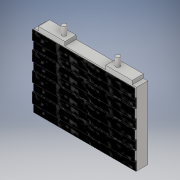
# Autodesk Inventor part: Cell
Saved by Autodesk Inventor 2017 (Build 210142000, 142)
## iProperties
Created: 2021-02-12
Part Number: Cell
Material: Generic
Document SubType Name: Modeling
Designer: Win240
Density: 1 g/cm^3
Appearance: Default
Author: Win240
Autodesk Inventor part; units mm, degrees
ref_plane "YZ Plane" through (0, 0, 0) normal (1, 0, 0) x (0, 1, 0)
ref_plane "XZ Plane" through (0, 0, 0) normal (0, 1, 0) x (-1, 0, 0)
ref_plane "XY Plane" through (0, 0, 0) normal (0, 0, 1) x (1, 0, 0)
sketch "Sketch1" plane through (0, 0, 0) normal (0, 0, 1) x (1, 0, 0)
  line L0 (-60.325, -42.8625) -> (60.325, -42.8625)
  line L1 (60.325, -42.8625) -> (60.325, 42.8625)
  line L2 (60.325, 42.8625) -> (-60.325, 42.8625)
  line L3 (-60.325, 42.8625) -> (-60.325, -42.8625)
  line L4 (-60.325, -42.8625) -> (60.325, 42.8625) construction
  line L5 (60.325, -42.8625) -> (-60.325, 42.8625) construction
  line L6 (-55.245, 42.8625) -> (-55.245, 47.3075)
  line L7 (-55.245, 47.3075) -> (-24.13, 47.3075)
  line L8 (-24.13, 47.3075) -> (-24.13, 42.8625)
  line L9 (24.13, 42.8625) -> (24.13, 47.3075)
  line L10 (24.13, 47.3075) -> (55.245, 47.3075)
  line L11 (55.245, 47.3075) -> (55.245, 42.8625)
  point P0 (0, 0)
  dimension "d0" = 120.65
  dimension "d1" = 85.725
  dimension "d2" = 4.445
  dimension "d3" = 5.08
  dimension "d4" = 5.08
  dimension "d5" = 31.115
  constraints: 24 end point, 4 point on line, 4 vertical, 2 collinear, 2 horizontal, 2 midpoint, 2 parallel, 1 perpendicular
  measures "d0" distance of L1.end L2.end
  measures "d1" distance of L2.end L0.start
  measures "d2" distance between parallel lines of L7 L2
  measures "d3" distance between parallel lines of L6 L3
  measures "d4" distance between parallel lines of L1 L11
  measures "d5" distance of L9.end L10.end
extrude "Extrusion1" add sketch "Sketch1" along normal blind 13.335
ref_plane "Work Plane1" through (-60.325, 57.1375, 0) normal (0, -1, 0) x (1, 0, 0)
sketch "Sketch2" plane through (-55.245, 47.3075, 0) normal (0, 1, 0) x (1, 0, 0)
  line L0 (31.115, 0) -> (31.115, -13.335) construction
  line L1 (79.375, 0) -> (79.375, -13.335) construction
  line L2 (31.115, -6.6675) -> (23.495, -6.6675) construction
  line L3 (79.375, -6.6675) -> (86.995, -6.6675) construction
  circle A0 centre (23.495, -6.6675) radius 2.5
  circle A1 centre (86.995, -6.6675) radius 2.5
  point P0 (55.245, 0)
  dimension "d8" = 63.5
  dimension "d9" = 5
  constraints: 4 end point, 2 centre point, 2 coincident, 2 horizontal, 2 midpoint, 1 collinear, 1 equal radius
  measures "d8" distance of L3.end L2.end
  measures "d9" diameter of A1
extrude "Extrusion2" add sketch "Sketch2" along normal up to surface (9.83 mm away)
sketch "Sketch3" plane through (60.325, -42.8625, 0) normal (1, 0, 0) x (0, 0, -1)
  line L0 (0, 0) -> (-13.335, 0) construction
  line L1 (-13.335, 0) -> (-13.335, 10.7156)
  line L2 (-13.335, 10.7156) -> (-14.985, 10.7156)
  line L3 (-14.985, 10.7156) -> (-14.985, 21.4313)
  line L4 (-14.985, 21.4313) -> (-13.335, 21.4313)
  line L5 (-13.335, 21.4313) -> (-13.335, 32.1469)
  line L6 (-13.335, 32.1469) -> (-14.985, 32.1469)
  line L7 (-14.985, 32.1469) -> (-14.985, 42.8625)
  line L8 (-14.985, 42.8625) -> (-13.335, 42.8625)
  line L9 (-13.335, 42.8625) -> (-13.335, 53.5781)
  line L10 (-13.335, 53.5781) -> (-14.985, 53.5781)
  line L11 (-14.985, 53.5781) -> (-14.985, 64.2938)
  line L12 (-14.985, 64.2938) -> (-13.335, 64.2938)
  line L13 (-13.335, 64.2938) -> (-13.335, 75.0094)
  line L14 (-13.335, 75.0094) -> (-14.985, 75.0094)
  line L15 (-14.985, 75.0094) -> (-14.985, 85.725)
  line L16 (-15.585, 85.725) -> (-15.585, 74.4094)
  line L17 (-15.585, 74.4094) -> (-13.935, 74.4094)
  line L18 (-13.935, 74.4094) -> (-13.935, 64.8938)
  line L19 (-13.935, 64.8938) -> (-15.585, 64.8938)
  line L20 (-15.585, 64.8938) -> (-15.585, 52.9781)
  line L21 (-15.585, 52.9781) -> (-13.935, 52.9781)
  line L22 (-13.935, 52.9781) -> (-13.935, 43.4625)
  line L23 (-13.935, 43.4625) -> (-15.585, 43.4625)
  line L24 (-15.585, 43.4625) -> (-15.585, 31.5469)
  line L25 (-15.585, 31.5469) -> (-13.935, 31.5469)
  line L26 (-13.935, 31.5469) -> (-13.935, 22.0313)
  line L27 (-13.935, 22.0313) -> (-15.585, 22.0313)
  line L28 (-15.585, 22.0313) -> (-15.585, 10.1156)
  line L29 (-15.585, 10.1156) -> (-13.935, 10.1156)
  line L30 (-13.935, 10.1156) -> (-13.935, 0)
  line L31 (0, 85.725) -> (-13.335, 85.725) construction
  line L32 (-13.335, 85.725) -> (-14.985, 85.725) construction
  line L33 (-13.935, 0) -> (-13.335, 0)
  line L34 (-14.985, 85.725) -> (-15.585, 85.725)
  point P0 (0, 42.8625)
  dimension "d14" = 2.25
  dimension "d15" = 0.6
  constraints: 66 end point, 12 collinear, 10 horizontal, 7 equal length, 2 vertical, 14 other
  measures "d14" distance between parallel lines of L13 L16
  measures "d15" distance between parallel lines of L16 L15
extrude "Extrusion3" add sketch "Sketch3" against normal up to surface (120.65 mm away) separate body
body "Solid1"
body "Solid2"
